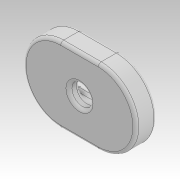
# Autodesk Inventor part: ValveThing
Saved by Autodesk Inventor 2020 (Build 240168000, 168)
## iProperties
Created: 2021-10-31
Part Number: ValveThing
Material: Generic
Document SubType Name: Modeling
Designer: DDeGo
Density: 1 g/cm^3
Appearance: Default
Author: DDeGo
Autodesk Inventor part; units mm, degrees
ref_plane "YZ Plane" through (0, 0, 0) normal (1, 0, 0) x (0, 1, 0)
ref_plane "XZ Plane" through (0, 0, 0) normal (0, 1, 0) x (-1, 0, 0)
ref_plane "XY Plane" through (0, 0, 0) normal (0, 0, 1) x (1, 0, 0)
sketch "Sketch1" plane through (0, 0, 0) normal (0, 0, 1) x (1, 0, 0)
  circle A0 centre (0, 0) radius 0.7
  line L0 (-1.25, 0) -> (1.25, 0) construction
  line L1 (-1.25, 2.5) -> (1.25, 2.5)
  line L2 (1.25, -2.5) -> (-1.25, -2.5)
  arc A1 (-1.25, 2.5) -> (-1.25, -2.5) centre (-1.25, 0) ccw
  arc A2 (1.25, -2.5) -> (1.25, 2.5) centre (1.25, 0) ccw
  dimension "d8" = 1.4
  dimension "d12" = 2.5
  dimension "d13" = 2.5
  constraints: 8 end point, 4 point on circle, 4 tangent, 3 centre point, 1 coincident, 1 horizontal, 1 midpoint, 1 parallel
  measures "d8" diameter of A0
  measures "d12" radius of A2
  measures "d13" distance of L0.start L0.end
extrude "Extrusion1" add sketch "Sketch1" along normal blind 1.4
sketch "Sketch3" plane through (0, 0, 0) normal (0, 0, -1) x (-1, 0, 0)
  arc A0 (1.25, -2.5) -> (1.25, 2.5) centre (1.25, 0) ccw projected
  line L0 (-1.25, 2.5) -> (1.25, 2.5) projected
  arc A1 (-1.25, 2.5) -> (-1.25, -2.5) centre (-1.25, 0) ccw projected
  line L1 (1.25, -2.5) -> (-1.25, -2.5) projected
  circle A2 centre (0, 0) radius 0.7 construction
  arc A3 (-1.25, 0.7) -> (-1.25, -0.7) centre (-1.25, 0) ccw
  line L2 (-1.25, 0.7) -> (1.25, 0.7)
  arc A4 (1.25, -0.7) -> (1.25, 0.7) centre (1.25, 0) ccw
  line L3 (1.25, -0.7) -> (-1.25, -0.7)
  circle A5 centre (0, 0) radius 0.7 construction
  constraints: 4 end point, 4 point on circle, 2 centre point, 1 tangent, 3 other
extrude "Extrusion3" cut sketch "Sketch3" against normal blind 0.7 contours L2 A4 L3 A3
fillet "Fillet1" radius 0.2 22 edges at (-0.7, 0, 1.4) (0.495, 0.495, 0.7) (0.495, -0.495, 0.7) (-0.7, 0, 0.7) (3.75, 0, 1.4) (0, 2.5, 1.4) (-3.75, 0, 1.4) (0, -2.5, 1.4) (3.75, 0, 0) (0, 2.5, 0) (-3.75, 0, 0) (0, -2.5, 0) (1.95, 0, 0) (0, 0.7, 0) (-1.95, 0, 0) (0, -0.7, 0) (-1.95, 0, 0.7) (-0.625, 0.7, 0.7) (-0.625, -0.7, 0.7) (1.95, 0, 0.7) (0.625, 0.7, 0.7) (0.625, -0.7, 0.7)
sketch "Sketch4" plane through (-1.25, -2.5, 0.2) normal (0, -1, 0) x (1, 0, 0)
  line L0 (2.5, 0) -> (2.5, 1) construction
  line L1 (2.5, 0.5) -> (0, 0.5) construction
  line L2 (0, 0) -> (0, 1) construction
  circle A0 centre (0, 0.5) radius 0.125
  circle A1 centre (0.625, 0.5) radius 0.125
  circle A2 centre (1.25, 0.5) radius 0.125
  circle A3 centre (1.875, 0.5) radius 0.125
  circle A4 centre (2.5, 0.5) radius 0.125
  point P0 (1.25, -0.2)
  dimension "d16" = 0.25
  dimension "d19" = 0.625
  constraints: 5 centre point, 2 coincident, 2 end point, 2 midpoint, 1 horizontal, 8 other
  measures "d16" diameter of A0
  measures "d19" distance of A0.centre A1.centre
extrude "Extrusion4" cut sketch "Sketch4" against normal blind 0.05 contours A2 | A3
body "Solid1"
